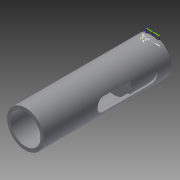
# Autodesk Inventor part: coverbody
Saved by Autodesk Inventor 2015 (Build 190159000, 159)
## iProperties
Created: 2014-11-30
Part Number: coverbody
Material: 常规
Document SubType Name: Modeling
Designer: zenkr
Density: 1 g/cm^3
Appearance: 默认
Author: zenkr
Autodesk Inventor part; units mm, degrees
ref_plane "XZ Plane" through (0, 0, 0) normal (0, 1, 0) x (-1, 0, 0)
ref_plane "XY Plane" through (0, 0, 0) normal (0, 0, 1) x (1, 0, 0)
sketch "草图1" plane through (0, 0, 0) normal (0, 1, 0) x (-1, 0, 0)
  circle A0 centre (0, 0) radius 5.5
  dimension "d0" = 11
  constraints: 1 centre point, 1 coincident
  measures "d0" diameter of A0
extrude "拉伸1" add sketch "草图1" along normal blind 38
sketch "草图2" plane through (0, 0, 0) normal (0, 1, 0) x (-1, 0, 0)
  circle A0 centre (0, 0) radius 4.5
  dimension "d3" = 9
  constraints: 1 centre point, 1 coincident
  measures "d3" diameter of A0
extrude "拉伸2" cut sketch "草图2" along normal blind 26.5
ref_plane "工作平面1" through (8, 0, 0) normal (1, 0, 0) x (0, 1, 0)
sketch "草图3" plane through (8, 0, 0) normal (1, 0, 0) x (0, 1, 0)
  line L0 (32, 0) -> (18, 0) construction
  line L1 (32, 2) -> (18, 2)
  line L2 (18, -2) -> (32, -2)
  arc A0 (32, -2) -> (32, 2) centre (32, 0) ccw
  arc A1 (18, 2) -> (18, -2) centre (18, 0) ccw
  line L3 (38, -5.5) -> (38, 5.5) projected
  line L4 (26.5, 2) -> (26.5, -2)
  point P0 (0, 0)
  point P1 (25, 0)
  dimension "d7" = 14
  dimension "d8" = 4
  dimension "d9" = 6
  dimension "d12" = 5.5
  constraints: 10 end point, 4 point on circle, 4 tangent, 2 centre point, 2 point on line, 1 horizontal, 1 midpoint, 1 parallel, 1 perpendicular
  measures "d7" distance of L0.start L0.end
  measures "d8" diameter of A1
  measures "d9" distance from line of L3 L0.start
  measures "d12" distance from line of L0.start L4
emboss "凸雕2" sketch "草图3" operation cut depth 0.5 direction (-1, 0, 0) contours A0 L2 L4 L1
extrude "拉伸3" cut sketch "草图3" against normal through all contours L4 L2 A1 L1
mirror "镜像1" about plane through (0, 0, 0) normal (1, 0, 0) of "凸雕2"
sketch "草图4" plane through (0, 38, 0) normal (0, 1, 0) x (1, 0, 0)
  arc A0 (2.6458, -3) -> (-2.6458, -3) centre (0, 0) ccw
  line L0 (-2.6458, -3) -> (2.6458, -3)
  point P0 (0, 4)
  dimension "d17" = 8
  dimension "d18" = 7
  constraints: 3 point on circle, 2 end point, 1 centre point, 1 coincident, 1 horizontal
  measures "d17" diameter of A0
  measures "d18" distance from line of L0 point (0, 4)
extrude "拉伸4" add sketch "草图4" along normal blind 0.5
fillet "圆角1" radius 0.4 2 edges at (0, 38.5, -4) (0, 38.5, 3) curvature continuous yes
sketch "草图5" plane through (0, 38, 0) normal (0, 1, 0) x (1, 0, 0)
  line L0 (2, -3.1) -> (-2, -3.1)
  line L1 (-2.6458, -3) -> (2.6458, -3) projected
  line L2 (0, 0) -> (0, -6.4081)
  line L3 (2, -3.1) -> (2, -6.106)
  line L4 (2, -6.106) -> (-2, -6.106)
  line L5 (-2, -6.106) -> (-2, -3.1)
  circle A0 centre (0, 0) radius 4.5 projected
  line L6 (2, -3.6) -> (-2, -3.6)
  point P0 (2, -4.0311)
  point P1 (-2, -4.0311)
  dimension "d22" = 4
  dimension "d23" = 0.1
  dimension "d30" = 0.5
  constraints: 12 end point, 4 point on line, 3 perpendicular, 2 point on circle, 2 vertical, 1 horizontal, 1 symmetric about line
  measures "d22" distance of L0.start L0.end
  measures "d23" distance between parallel lines of L1 L0
  measures "d30" distance between parallel lines of L0 L6
extrude "拉伸8" cut sketch "草图5" against normal blind 0.5 contours L3 L6 L2 L0 | L2 L6 L5 L0 | L3 A0 L2 L6 | L2 A0 L5 L6 | L3 L4 L2 A0 | L2 L4 L5 A0
extrude "拉伸9" cut sketch "草图5" against normal blind 4.5 contours L3 L6 L2 L0 | L2 L6 L5 L0
